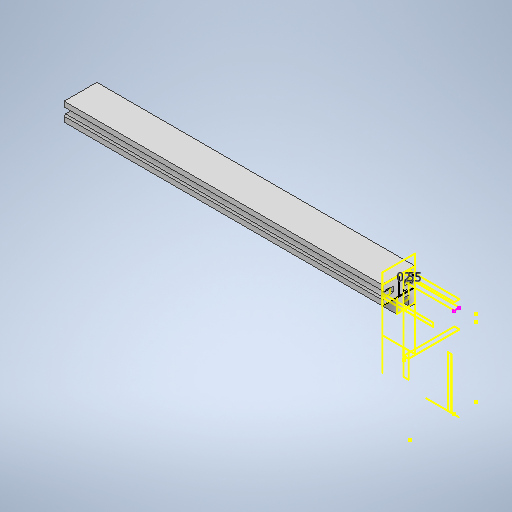
# Autodesk Inventor part: Kątownikśrodek x 3
Saved by Autodesk Inventor 2025 (Build 290162000, 162)
## iProperties
Created: 2025-07-31
Part Number: Kątownikśrodek x 3
Material: Ogólny
Document SubType Name: Modeling
Designer: ThePi
Density: 1 g/cm^3
Appearance: Domyślna
Author: ThePi
Autodesk Inventor part; units mm, degrees
ref_plane "YZ Plane" through (0, 0, 0) normal (1, 0, 0) x (0, 1, 0)
ref_plane "XZ Plane" through (0, 0, 0) normal (0, 1, 0) x (-1, 0, 0)
ref_plane "XY Plane" through (0, 0, 0) normal (0, 0, 1) x (1, 0, 0)
derived "2xKątownik.ipt"
sketch "Szkic33" plane through (-49.25, 0, -7.5) normal (-1, 0, 0) x (0, 0, 1)
  line L0 (4.5, 31) -> (3.5, 30) projected
  line L1 (4.5, 31) -> (4.5, 35) projected
  line L2 (4.5, 35) -> (8, 35) projected
  line L3 (8, 35) -> (8, 31) projected
  line L4 (9, 30) -> (8, 31) projected
  line L5 (9, 30) -> (12.5, 30) projected
  line L6 (12.5, 30) -> (12.5, 40) projected
  line L7 (12.5, 40) -> (22.5, 40) projected
  line L8 (22.5, 43.5) -> (22.5, 40) projected
  line L9 (21.5, 44.5) -> (22.5, 43.5) projected
  line L10 (21.5, 44.5) -> (17.5, 44.5) projected
  line L11 (17.5, 44.5) -> (17.5, 48) projected
  line L12 (17.5, 48) -> (21.5, 48) projected
  line L13 (22.5, 49) -> (21.5, 48) projected
  line L14 (22.5, 52.5) -> (22.5, 49) projected
  line L15 (22.5, 52.5) -> (9, 52.5) projected
  line L16 (8, 51.5) -> (9, 52.5) projected
  line L17 (8, 51.5) -> (8, 47.5) projected
  line L18 (8, 47.5) -> (4.5, 47.5) projected
  line L19 (4.5, 47.5) -> (4.5, 51.5) projected
  line L20 (3.5, 52.5) -> (4.5, 51.5) projected
  line L21 (3.5, 52.5) -> (0, 52.5) projected
  line L22 (0, 52.5) -> (0, 30) projected
  line L23 (0, 30) -> (3.5, 30) projected
  point P0 (7.5, 0)
extrude "Wyciągnięcie proste1" add sketch "Szkic33" along normal blind 219
sketch "Szkic19" plane through (-49.25, 30, -7.5) normal (1, 0, 0) x (0, 0, -1)
  line L0 (-9, 22.5) -> (-8, 21.5) projected
  line L1 (-8, 5) -> (-8, 22.5) projected
  line L2 (-4.5, 17.5) -> (-8, 17.5) projected
  line L3 (-4.5, 5) -> (-4.5, 22.5) projected
  line L4 (-4.5, 21.5) -> (-3.5, 22.5) projected
  line L5 (-3.5, 22.5) -> (0, 22.5) projected
  line L6 (-9, 22.5) -> (-3.5, 22.5)
  point P0 (-7.5, -30)
  constraints: 2 end point, 1 horizontal
extrude "Wyciągnięcie proste2" add sketch "Szkic19" against normal up to surface (219 mm away)
sketch "Szkic20" plane through (-49.25, 30, -7.5) normal (1, 0, 0) x (0, 0, -1)
  line L0 (-22.5, 22.5) -> (0, 22.5) projected
  line L1 (0, 22.5) -> (-22.5, 22.5)
  line L2 (-22.5, 19) -> (-22.5, 22.5) projected
  line L3 (-22.5, 22.5) -> (-22.5, 19)
  line L4 (-21.5, 18) -> (-22.5, 19) projected
  line L5 (-22.5, 19) -> (-21.5, 18)
  line L6 (-17.5, 14.5) -> (-17.5, 18) projected
  line L7 (-21.5, 18) -> (-17.5, 18)
  line L8 (-17.5, 18) -> (-17.5, 14.5)
  line L9 (-21.5, 14.5) -> (-17.5, 14.5) projected
  line L10 (-17.5, 14.5) -> (-21.5, 14.5)
  line L11 (-21.5, 14.5) -> (-22.5, 13.5)
  line L12 (-22.5, 10) -> (-22.5, 13.5) projected
  line L13 (-22.5, 13.5) -> (-22.5, 10)
  line L14 (-12.5, 0) -> (-12.5, 10) projected
  line L15 (-22.5, 10) -> (-12.5, 10)
  line L16 (-12.5, 10) -> (0, 10)
  line L17 (0, 10) -> (0, 22.5)
  line L18 (-22.5, 22.5) -> (-11.25, 22.5)
  line L19 (-11.25, 10) -> (-11.25, 22.5)
  line L20 (0, 22.5) -> (-22.5, 22.5)
  line L21 (0, 19) -> (0, 22.5)
  line L22 (-1, 18) -> (0, 19)
  line L23 (-5, 14.5) -> (-5, 18)
  line L24 (-1, 18) -> (-5, 18)
  line L25 (-1, 14.5) -> (-5, 14.5)
  line L26 (-1, 14.5) -> (0, 13.5)
  line L27 (0, 10) -> (0, 13.5)
  line L28 (0, 10) -> (-10, 10)
  line L29 (-10, 10) -> (-22.5, 10)
  line L30 (0, 19) -> (0, 13.5)
  line L31 (-1, 14.5) -> (-5, 14.5)
  line L32 (-5, 14.5) -> (-5, 18)
  line L33 (-5, 18) -> (-1, 18)
  line L34 (-1, 18) -> (0, 19)
  line L35 (-1, 14.5) -> (0, 13.5)
  line L36 (-5, 18) -> (-5, 17.5)
  line L37 (-5, 17.5) -> (0, 17.5)
  line L38 (0, 17.5) -> (0, 15)
  line L39 (0, 15) -> (-5, 15)
  line L40 (-5, 15) -> (-5, 17.5)
  line L41 (0, 17.5) -> (0, 15)
  point P0 (-7.5, -30)
  point P1 (0, 15)
  point P2 (0, 17.5)
  point P3 (-5, 17.5)
  dimension "d7" = 0.5
  dimension "d8" = 2.5
  constraints: 70 end point, 11 symmetric about line, 10 perpendicular, 8 collinear, 8 point on line, 1 horizontal, 1 midpoint, 1 parallel
  measures "d7" distance of L24.end L36.end
  measures "d8" distance of L37.end L38.end
extrude "Wyciągnięcie proste4" cut sketch "Szkic20" against normal up to surface (219 mm away) contours L17 L37 L23 L24 L22 | L17 L39 L23 L37 | L17 L26 L25 L23 L39
thicken "Pogrubienie1" operation cut thickness 2.5 both sides no extend neighbours no toward (0, 0, 1) faces at (-122.25, 46.8333, -2.5)
thicken "Pogrubienie2" operation cut thickness 2.5 both sides no extend neighbours no toward (0, 0, -1) faces at (-122.25, 45.6667, 10)
thicken "Pogrubienie3" operation cut thickness 2.5 both sides no extend neighbours no toward (0, 1, 0) faces at (-122.25, 35, -1.8333)
sketch "Szkic3" plane through (0, 0, 0) normal (0, -1, 0) x (1, 0, 0)
  point P0 (0, 0)
sketch "Szkic8" plane through (-49.25, 0, -7.5) normal (-1, 0, 0) x (0, 0, 1)
  point P0 (7.5, 0)
sketch "Szkic9" plane through (0, 0, 0) normal (0, -1, 0) x (1, 0, 0)
  point P0 (0, 0)
sketch "Szkic10" plane through (-49.25, 0, -7.5) normal (-1, 0, 0) x (0, 0, 1)
  line L0 (0, 0) -> (0, 60) projected
  line L1 (0, 30) -> (0, 52.5) projected
  line L2 (0, 52.5) -> (22.5, 52.5) projected
  line L3 (22.5, 0) -> (22.5, 60) projected
  line L4 (22.5, 52.5) -> (22.5, 40) projected
  line L5 (22.5, 40) -> (12.5, 40) projected
  line L6 (12.5, 40) -> (12.5, 30) projected
  line L7 (0, 30) -> (5, 30) projected
  line L8 (12.5, 30) -> (0, 30) projected
  line L9 (22.5, 52.5) -> (22.5, 60) projected
  line L10 (22.5, 60) -> (0, 60) projected
  line L11 (0, 60) -> (0, 52.5) projected
  line L12 (22.5, 52.5) -> (0, 52.5) projected
  point P0 (7.5, 0)
sketch "Szkic11" plane through (0, 0, 0) normal (0, -1, 0) x (1, 0, 0)
  point P0 (0, 0)
sketch "Szkic15" plane through (-1.75, 0, 15) normal (0, 0, 1) x (1, 0, 0)
  line L0 (0, 0) -> (0, 30) projected
  line L1 (0, 0) -> (0, 35) projected
  line L2 (0, 35) -> (0, 0) projected
  line L3 (-2.5, 0) -> (-2.5, 30) projected
  line L4 (0, 0) -> (-2.5, 0) projected
  line L5 (5, 0) -> (-17.5, 0) projected
  line L6 (-2.5, 0) -> (-2.5, 35) projected
  line L7 (-2.5, 35) -> (0, 35) projected
  line L8 (0, 0) -> (0, 35) projected
  line L9 (-17.5, 45) -> (-47.5, 45) projected
  line L10 (-47.5, 45) -> (-12.5, 45) projected
  line L11 (-12.5, 45) -> (-47.5, 45) projected
  line L12 (-47.5, 47.5) -> (-17.5, 47.5) projected
  line L13 (-47.5, 45) -> (-47.5, 47.5) projected
  line L14 (-47.5, 47.5) -> (-12.5, 47.5) projected
  line L15 (-12.5, 47.5) -> (-12.5, 45) projected
  point P0 (1.75, 0)
sketch "Szkic21" plane through (-49.25, 0, -7.5) normal (-1, 0, 0) x (0, 0, 1)
  line L0 (4.5, 35) -> (8, 35) projected
  line L1 (4.5, 35) -> (4.5, 52.5) projected
  line L2 (22.5, 52.5) -> (0, 52.5) projected
  line L3 (8, 0) -> (8, 35) projected
  line L4 (8, 35) -> (8, 52.5) projected
  line L5 (8, 52.5) -> (4.5, 52.5) projected
  line L6 (4.5, 52.5) -> (4.5, 47.5) projected
  line L7 (4.5, 47.5) -> (8, 47.5) projected
  point P0 (7.5, 0)
sketch "Szkic22" plane through (-9.25, 0, 45) normal (0, 0, 1) x (1, 0, 0)
  point P0 (9.25, 0)
sketch "Szkic23" plane through (-9.25, 0, 45) normal (0, 0, 1) x (1, 0, 0)
  line L0 (4.5, 35) -> (8, 35) projected
  line L1 (4.5, 35) -> (4.5, 52.5) projected
  line L2 (12.5, 52.5) -> (-10, 52.5) projected
  line L3 (8, 35) -> (8, 52.5) projected
  line L4 (8, 52.5) -> (4.5, 52.5) projected
  line L5 (4.5, 52.5) -> (4.5, 47.5) projected
  line L6 (4.5, 47.5) -> (8, 47.5) projected
  point P0 (9.25, 0)
sketch "Szkic25" plane through (-49.25, 52.5, -7.5) normal (0, 1, 0) x (1, 0, 0)
  line L0 (0, -8) -> (0, -4.5) projected
  line L1 (0, -4.5) -> (0, -8) projected
  line L2 (0, -8) -> (35, -8) projected
  line L3 (35, -8) -> (35, -4.5) projected
  line L4 (35, -4.5) -> (0, -4.5) projected
  point P0 (49.25, -7.5)
sketch "Szkic27" plane through (-4.75, 47.5, 45) normal (0, 1, 0) x (1, 0, 0)
  line L0 (3.5, 35) -> (0, 35) projected
  line L1 (-14.5, 48) -> (-44.5, 48) projected
  line L2 (-44.5, 48) -> (-44.5, 44.5) projected
  line L3 (-44.5, 48) -> (-44.5, 44.5) projected
  line L4 (-9.5, 48) -> (-9.5, 44.5) projected
  line L5 (-44.5, 44.5) -> (-9.5, 44.5) projected
  line L6 (-9.5, 44.5) -> (-9.5, 48) projected
  line L7 (-9.5, 48) -> (-44.5, 48.1482) projected
  line L8 (3.5, 0) -> (3.5, 35) projected
  line L9 (3.5, 0) -> (0, 0) projected
  line L10 (3.5, 0) -> (0, 0) projected
  line L11 (0, 0) -> (0, 35) projected
  line L12 (0, 35) -> (3.5, 35) projected
  line L13 (3.5, 0) -> (3.5, 35) projected
  point P0 (4.75, 45)
